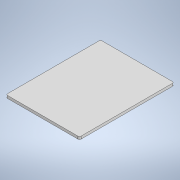
# Autodesk Inventor part: ur3_base
Saved by Autodesk Inventor 2022 (Build 260153000, 153)
## iProperties
Created: 2022-08-11
Part Number: ur3_base
Material: Generic
Document SubType Name: Modeling
Designer: Alok
Density: 1 g/cm^3
Appearance: Default
Author: Alok
Autodesk Inventor part; units mm, degrees
ref_plane "YZ Plane" through (0, 0, 0) normal (1, 0, 0) x (0, 1, 0)
ref_plane "XZ Plane" through (0, 0, 0) normal (0, 1, 0) x (-1, 0, 0)
ref_plane "XY Plane" through (0, 0, 0) normal (0, 0, 1) x (1, 0, 0)
sketch "Sketch1" plane through (0, 0, 0) normal (0, 1, 0) x (-1, 0, 0)
  line L0 (70, 90) -> (-70, 90)
  line L1 (-70, 90) -> (-70, -90)
  line L2 (-70, -90) -> (70, -90)
  line L3 (70, -90) -> (70, 90)
  line L4 (70, 90) -> (-70, -90) construction
  line L5 (-70, 90) -> (70, -90) construction
  point P0 (0, 0)
  dimension "d0" = 140
  dimension "d1" = 180
  constraints: 12 end point, 2 midpoint, 2 parallel, 1 horizontal, 1 perpendicular
  measures "d0" distance of L2.end L1.end
  measures "d1" distance of L1.end L0.end
extrude "Extrusion1" add sketch "Sketch1" along normal blind 5
fillet "Face Fillet1" radius 3 1 edges at (70, 2.5, 90)
fillet "Face Fillet2" radius 3 1 edges at (70, 2.5, -90)
fillet "Face Fillet3" radius 3 1 edges at (-70, 2.5, -90)
fillet "Face Fillet4" radius 3 1 edges at (-70, 2.5, 90)
body "Solid1"
